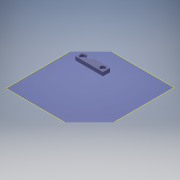
# Autodesk Inventor part: 21_Z-Focus_Halterung
Saved by Autodesk Inventor 2016 (Build 200138000, 138)
## iProperties
Created: 2016-09-11
Part Number: 21_Z-Focus_Halterung
Material: Generisch
Document SubType Name: Modeling
Designer: Bene
Density: 1 g/cm^3
Appearance: Vorgabe
Author: Bene
Autodesk Inventor part; units mm, degrees
ref_plane "YZ Plane" through (0, 0, 0) normal (1, 0, 0) x (0, 1, 0)
ref_plane "XZ Plane" through (0, 0, 0) normal (0, 1, 0) x (-1, 0, 0)
ref_plane "XY Plane" through (0, 0, 0) normal (0, 0, 1) x (1, 0, 0)
ref_plane "Arbeitsebene2" through (22.407, -67.7758, 25.2477) normal (0, 0, -1) x (0, 1, 0)
sketch "Skizze2" plane through (22.407, -67.7758, 25.2477) normal (0, 0, -1) x (0, 1, 0)
  circle A0 centre (39.5, -18.5) radius 2.5 construction
  circle A1 centre (39.5, -52) radius 2.5 construction
  circle A2 centre (46, -45) radius 4 construction
  arc A3 (-61, 63) -> (-64, 60) centre (-61, 60) ccw construction
  line L0 (-64, 60) -> (-64, -60) construction
  arc A4 (-64, -60) -> (-61, -63) centre (-61, -60) ccw construction
  line L1 (-61, -63) -> (52, -63) construction
  arc A5 (52, -63) -> (55, -60) centre (52, -60) ccw construction
  line L2 (55, -60) -> (55, -8.8167) construction
  arc A6 (57.4545, -5.8667) -> (55, -8.8167) centre (58, -8.8167) ccw construction
  arc A7 (57.4545, -5.8667) -> (64, 2) centre (56, 2) ccw construction
  line L3 (64, 2) -> (64, 60) construction
  arc A8 (64, 60) -> (61, 63) centre (61, 60) ccw construction
  line L4 (61, 63) -> (-61, 63) construction
  line L5 (33.5, -58) -> (45.5, -58)
  line L6 (45.5, -58) -> (45.5, -12)
  line L7 (45.5, -12) -> (33.5, -12)
  line L8 (33.5, -12) -> (33.5, -58)
  circle A9 centre (46, -45) radius 5.5
  circle A10 centre (39.5, -52) radius 4.0525
  circle A11 centre (39.5, -18.5) radius 4.0525
  line L9 (45.5, -22.407) -> (45.5, -37.7678)
  point P0 (45.5, -50.4772)
  point P1 (45.5, -39.5228)
  dimension "d2" = 12
  dimension "d3" = 46
  dimension "d4" = 6
  dimension "d5" = 6
  dimension "d6" = 11
  constraints: 10 end point, 3 centre point, 3 coincident, 3 point on line, 2 parallel, 2 point on circle, 1 horizontal, 1 perpendicular, 1 tangent
  measures "d2" distance of L7.end L6.end
  measures "d3" distance of L6.end L5.end
  measures "d4" distance from line of A1.centre L5
  measures "d5" distance from line of L8 A1.centre
  measures "d6" diameter of A9
extrude "Extrusion2" add sketch "Skizze2" along normal blind 4 contours L8 L7 L6 A9 L5
sketch "Skizze3" plane through (22.407, -67.7758, 21.2477) normal (0, 0, -1) x (-1, 0, 0)
  circle A0 centre (18.5, 39.5) radius 4.0525 projected
  line L0 (58, 45.5) -> (50.4772, 45.5) projected
  line L1 (12, 45.5) -> (12, 33.5) projected
  line L2 (12, 33.5) -> (58, 33.5) projected
  line L3 (58, 33.5) -> (58, 45.5) projected
  arc A1 (49.0304, 42.2575) -> (50.4772, 45.5) centre (45, 46) ccw projected
  circle A2 centre (52, 39.5) radius 4.0525 projected
  arc A3 (39.5228, 45.5) -> (49.0304, 42.2575) centre (45, 46) ccw projected
  circle A4 centre (18.5, 39.5) radius 1.5 projected
  circle A5 centre (52, 39.5) radius 1.5 projected
  line L4 (39.5228, 45.5) -> (12, 45.5) projected
  point P0 (22.407, 67.7758)
  constraints: 1 other
extrude "Extrusion3" add sketch "Skizze3" along normal blind 2 contours A0 | A2 | L3 L2 L1 L4 A3 A1 L0
sketch "Skizze9" plane through (-17.1158, -22.2758, 25.2477) normal (0, 1, 0) x (1, 0, 0)
  line L0 (0, 0) -> (27.5228, 0) projected
  line L1 (27.5228, 0) -> (27.5228, 6) projected
  line L2 (0, 6) -> (27.5228, 6) projected
  line L3 (0, 0) -> (0, 6) projected
  point P0 (17.1158, 25.2477)
ref_plane "Arbeitsebene4" through (-14.093, -4, 15.1634) normal (0, -1, 0) x (0, 0, -1)
sketch "Skizze10" plane through (-14.093, -4, 15.1634) normal (0, -1, 0) x (0, 0, -1)
  circle A0 centre (-0.3366, 0) radius 2.5 projected
  line L0 (-5, -15) -> (-5, 15) projected
  line L1 (5, -15) -> (-5, -15) projected
  line L2 (5, 15) -> (5, -15) projected
  line L3 (-5, 15) -> (5, 15) projected
  point P0 (15.1634, 14.093)
extrude "Extrusion5" add sketch "Skizze10" along normal blind 1
sketch "Skizze11" plane through (-14.093, -5, 15.1634) normal (0, -1, 0) x (1, 0, 0)
  circle A0 centre (0, 0.3366) radius 2.5 projected
  line L0 (15, 5) -> (-15, 5) projected
  line L1 (-15, 5) -> (-15, -5) projected
  line L2 (-15, -5) -> (15, -5) projected
  line L3 (15, -5) -> (15, 5) projected
  point P0 (14.093, -15.1634)
